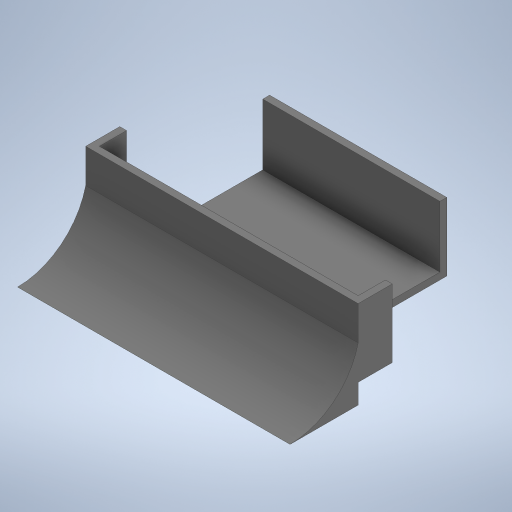
# Autodesk Inventor part: intro 2 robot
Saved by Autodesk Inventor 2024.4 (Build 284460000, 460)
## iProperties
Created: 2025-11-27
Part Number: intro 2 robot
Material: Generic
Document SubType Name: Modeling
Designer: hp
Density: 1 g/cm^3
Appearance: Default
Author: hp
Autodesk Inventor part; units mm, degrees
ref_plane "YZ Plane" through (0, 0, 0) normal (1, 0, 0) x (0, 1, 0)
ref_plane "XZ Plane" through (0, 0, 0) normal (0, 1, 0) x (-1, 0, 0)
ref_plane "XY Plane" through (0, 0, 0) normal (0, 0, 1) x (1, 0, 0)
sketch "Sketch6" plane through (0, 0, 0) normal (1, 0, 0) x (0, 1, 0)
  line L0 (0, 0) -> (0, 100)
  line L1 (0, 100) -> (50, 100)
  line L2 (50, 100) -> (50, 95)
  line L3 (50, 95) -> (5, 95)
  line L4 (5, 95) -> (5, 5)
  line L5 (5, 5) -> (50, 5)
  line L6 (50, 5) -> (50, 0)
  line L7 (50, 0) -> (0, 0)
  line L8 (0, 100) -> (-14.5, 100)
  line L9 (-14.5, 100) -> (-14.5, 150)
  arc A0 (-14.5, 150) -> (25, 100) centre (36.8956, 150) ccw
  dimension "d66" = 14.5
  dimension "d67" = 50
  dimension "d68" = 50
  dimension "d69" = 45
  dimension "d87" = 90
  constraints: 20 end point, 6 perpendicular, 2 point on circle, 2 point on line, 2 vertical, 1 centre point, 1 horizontal, 1 midpoint, 1 tangent
  measures "d66" distance of L0.end L8.end
  measures "d67" distance of L8.end L9.end
  measures "d68" distance of L6.end L0.start
  measures "d69" distance of L4.end L5.end
  measures "d87" distance between parallel lines of L5 L3
extrude "Extrusion6" add sketch "Sketch6" along normal blind 200
sketch "Sketch7" plane through (0, 5, 95) normal (0, 0, -1) x (-1, 0, 0)
  line L0 (0, 45) -> (-200, 45) projected
  line L1 (0, 0) -> (-200, 0) projected
  line L2 (-200, 45) -> (-195, 45)
  line L3 (-195, 45) -> (-195, 0)
  line L4 (-195, 0) -> (-200, 0)
  line L5 (-200, 0) -> (-200, 45)
  point P0 (0, -5)
  dimension "d52" = 5
  constraints: 8 end point, 2 parallel, 1 horizontal, 1 perpendicular, 1 point on line
  measures "d52" distance of L3.end L4.end
extrude "Extrusion7" add sketch "Sketch7" along normal blind 90
sketch "Sketch8" plane through (0, 5, 95) normal (0, 0, -1) x (-1, 0, 0)
  line L0 (0, 45) -> (-195, 45) projected
  line L1 (0, 0) -> (-195, 0) projected
  line L2 (0, 45) -> (-5, 45)
  line L3 (-5, 45) -> (-5, 0)
  line L4 (-5, 0) -> (0, 0)
  line L5 (0, 0) -> (0, 45)
  point P0 (0, -5)
  dimension "d55" = 5
  constraints: 8 end point, 2 parallel, 1 horizontal, 1 perpendicular, 1 point on line
  measures "d55" distance of L4.end L3.end
extrude "Extrusion8" add sketch "Sketch8" along normal blind 90
sketch "Sketch9" plane through (200, 0, 0) normal (1, 0, 0) x (0, 0, -1)
  line L0 (0, 0) -> (0, 50) projected
  line L1 (-100, 0) -> (0, 0) projected
  line L2 (0, 50) -> (-75, 50)
  line L3 (-75, 50) -> (-75, 0)
  line L4 (-75, 0) -> (0, 0)
  line L5 (0, 0) -> (0, 50)
  circle A0 centre (-35, 18) radius 33.5
  dimension "d95" = 75
  dimension "d96" = 67
  constraints: 8 end point, 2 parallel, 1 centre point, 1 horizontal, 1 perpendicular, 1 point on line
  measures "d95" distance of L4.end L3.end
  measures "d96" diameter of A0
extrude "Extrusion9" cut sketch "Sketch9" against normal blind 35 contours L1 A0 L2 L0 | L1 A0 L2 | L1 L3 L2 A0
sketch "Sketch10" plane through (0, 0, 0) normal (-1, 0, 0) x (0, 0, 1)
  line L0 (0, 50) -> (100, 50) projected
  line L1 (100, 0) -> (0, 0) projected
  line L2 (0, 50) -> (75, 50)
  line L3 (75, 50) -> (75, 0)
  line L4 (75, 0) -> (0, 0)
  line L5 (0, 0) -> (0, 50)
  circle A0 centre (35, 18) radius 33.5
  dimension "d94" = 75
  dimension "d97" = 67
  constraints: 8 end point, 2 parallel, 1 centre point, 1 horizontal, 1 perpendicular, 1 point on line
  measures "d94" distance of L3.end L4.end
  measures "d97" diameter of A0
extrude "Extrusion10" cut sketch "Sketch10" against normal blind 35 contours L0 A0 L1 L5 | L0 A0 L1 | L0 L3 L1 A0
body "Solid3"
